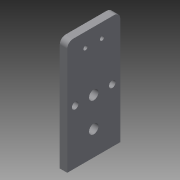
# Autodesk Inventor part: carriage
Saved by Autodesk Inventor 2015 SP1 (Build 190203100, 203)
## iProperties
Created: 2016-07-08
Part Number: carriage
Material: Generic
Document SubType Name: Modeling
Designer: lustinga
Density: 1 g/cm^3
Appearance: Default
Mass: 11.2089 g
Surface Area: 81.0297 cm^2
Volume: 11.2089 cm^3
Author: lustinga
Autodesk Inventor part; units mm, degrees
ref_plane "YZ Plane" through (0, 0, 0) normal (1, 0, 0) x (0, 1, 0)
ref_plane "XZ Plane" through (0, 0, 0) normal (0, 1, 0) x (-1, 0, 0)
ref_plane "XY Plane" through (0, 0, 0) normal (0, 0, 1) x (1, 0, 0)
sketch "Sketch1" plane through (0, 0, 0) normal (1, 0, 0) x (0, 1, 0)
  line L0 (-16.0539, 66.6862) -> (18.9461, 66.6862)
  line L1 (23.9461, 61.6862) -> (23.9461, -29.3138)
  line L2 (-21.0539, -29.3138) -> (-21.0539, 61.6862)
  circle A0 centre (-6.3039, -8.3138) radius 1.75
  circle A1 centre (1.4461, -16.0638) radius 1.75
  circle A2 centre (9.1961, -8.3138) radius 1.75
  circle A3 centre (1.4461, -0.5638) radius 1.75
  circle A4 centre (1.4461, 16.6862) radius 4
  line L3 (-21.0539, -29.3138) -> (23.9461, -29.3138)
  circle A5 centre (17.1961, 16.6862) radius 2.8
  circle A6 centre (1.4461, -8.3138) radius 4
  circle A7 centre (-14.3039, 16.6862) radius 2.8
  arc A8 (-16.0539, 66.6862) -> (-21.0539, 61.6862) centre (-16.0539, 61.6862) ccw
  arc A9 (23.9461, 61.6862) -> (18.9461, 66.6862) centre (18.9461, 61.6862) ccw
  circle A10 centre (-5.5539, 56.6862) radius 1.75
  circle A11 centre (8.4461, 56.6862) radius 1.75
  point P0 (0, 0)
  point P1 (-21.0539, 66.6862)
  point P2 (23.9461, 66.6862)
  dimension "d4" = 360
  dimension "d7" = 8
  dimension "d15" = 8
  dimension "d16" = 5.6
  dimension "d20" = 5.6
  dimension "d21" = 31.5
  dimension "d22" = 15.75
  dimension "d23" = 25
  dimension "d25" = 5
  dimension "d26" = 45
  dimension "d28" = 22.5
  dimension "d29" = 14
  dimension "d30" = 15.5
  dimension "d31" = 3.5
  dimension "d32" = 3.5
  dimension "d33" = 91
  dimension "d34" = 10
  constraints: 12 centre point, 8 end point, 4 point on circle, 4 point on line, 4 tangent, 1 coincident, 1 equal radius, 1 horizontal, 1 parallel, 1 perpendicular, 9 other
  measures "d7" diameter of A4
  measures "d15" diameter of A6
  measures "d16" diameter of A5
  measures "d20" diameter of A7
  measures "d21" distance of A5.centre A7.centre
  measures "d22" distance of A4.centre A5.centre
  measures "d23" distance of A6.centre A4.centre
  measures "d25" radius of A8
  measures "d26" distance of L2.start L1.end
  measures "d28" distance from line of L1 A4.centre
  measures "d29" distance of A11.centre A10.centre
  measures "d30" distance from line of L2 A10.centre
  measures "d31" diameter of A10
  measures "d32" diameter of A11
  measures "d33" distance of L2.start L2.end
  measures "d34" distance from line of L0 A10.centre
extrude "Extrusion1" add sketch "Sketch1" along normal blind 6.35 contours L0 A9 L1 L3 L2 A8 | A0 | A1 | A2 | A3
equation "\"d28\" = 0.5 * d26"
body "Solid1"
